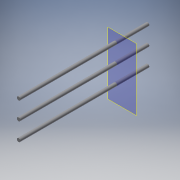
# Autodesk Inventor part: Rails
Saved by Autodesk Inventor 2016 (Build 200138000, 138)
## iProperties
Created: 2016-04-17
Part Number: Rails
Material: Generic
Document SubType Name: Modeling
Designer: Scott
Density: 1 g/cm^3
Appearance: Default
Author: Scott
Autodesk Inventor part; units mm, degrees
ref_plane "YZ Plane" through (0, 0, 0) normal (1, 0, 0) x (0, 1, 0)
ref_plane "XZ Plane" through (0, 0, 0) normal (0, 1, 0) x (-1, 0, 0)
ref_plane "XY Plane" through (0, 0, 0) normal (0, 0, 1) x (1, 0, 0)
ref_plane "Work Plane1" through (-2.9808, 6.4412, -99.06) normal (0, 0, -1) x (-1, 0, 0)
sketch "Sketch1" plane through (-2.9808, 6.4412, -99.06) normal (0, 0, -1) x (-1, 0, 0)
  line L0 (-33.4608, 12.473) -> (-25.4659, 12.473) projected
  line L1 (-25.4659, 12.473) -> (-25.4659, 7.473) projected
  line L2 (-25.4659, 7.473) -> (-20.4659, 12.473) projected
  line L3 (-20.4659, 12.473) -> (-11.4709, 12.473) projected
  line L4 (-11.4709, 12.473) -> (-11.4709, 4.473) projected
  line L5 (-17.4709, 4.473) -> (-11.4709, 4.473) projected
  line L6 (-17.4709, -1.527) -> (-17.4709, 4.473) projected
  line L7 (-11.4709, -1.527) -> (-17.4709, -1.527) projected
  line L8 (-11.4709, -1.527) -> (-11.4709, -9.527) projected
  line L9 (-11.4709, -9.527) -> (-20.4659, -9.527) projected
  line L10 (-20.4659, -9.527) -> (-25.4659, -4.527) projected
  line L11 (-25.4659, -4.527) -> (-25.4659, -9.527) projected
  line L12 (-25.4659, -9.527) -> (-33.4608, -9.527) projected
  line L13 (-33.4608, -9.527) -> (-33.4608, -37.1779) projected
  line L14 (-33.4608, -37.1779) -> (27.4992, -72.3732) projected
  line L15 (27.4992, -72.3732) -> (27.4992, 59.4908) projected
  line L16 (27.4992, 59.4908) -> (-33.4608, 59.4908) projected
  line L17 (-33.4608, 59.4908) -> (-33.4608, 12.473) projected
  circle A0 centre (13.0324, -40.4049) radius 8 projected
  circle A1 centre (13.0324, 43.3508) radius 8 projected
  circle A2 centre (13.0324, 1.473) radius 11.5 projected
  circle A3 centre (13.0324, 43.3508) radius 4
  circle A4 centre (13.0324, 1.473) radius 4
  circle A5 centre (13.0324, -40.4049) radius 4
  line L18 (-25.4659, 12.473) -> (-20.4659, 12.473)
  line L19 (-12.9659, -8.527) -> (-32.9659, -8.527)
  line L20 (-32.9659, -8.527) -> (-32.9659, 11.473)
  line L21 (-32.9659, 11.473) -> (-12.9659, 11.473)
  line L22 (-12.9659, 11.473) -> (-12.9659, -8.527)
  line L23 (-12.9659, -8.527) -> (-32.9659, 11.473) construction
  line L24 (-32.9659, -8.527) -> (-12.9659, 11.473) construction
  point P0 (-2.9808, -6.4412)
  point P1 (-22.9659, 1.473)
  dimension "d0" = 8
  dimension "d1" = 8
  dimension "d2" = 8
  dimension "d7" = 20
  dimension "d8" = 20
  constraints: 14 end point, 3 centre point, 3 coincident, 2 horizontal, 2 midpoint, 2 parallel, 1 perpendicular
  measures "d0" diameter of A3
  measures "d1" diameter of A4
  measures "d2" diameter of A5
  measures "d7" distance of L20.end L21.end
  measures "d8" distance of L19.end L20.end
extrude "Extrusion1" add sketch "Sketch1" along normal blind 75 and the other way blind 225 contours L21 L2 L1 | L1 L2 L21 L22 L5 L6 L7 L19 L10 L11 L20 | L11 L10 L19 | L22 L7 L6 L5 | A3 | A4 | A5
body "Solid1"
